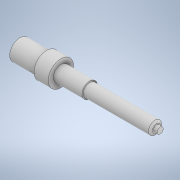
# Autodesk Inventor part: Eixo caixa de engrenagem
Saved by Autodesk Inventor 2022.1 (Build 261234020, 234B)
## iProperties
Created: 2023-11-06
Part Number: Eixo caixa de engrenagem
Material: Generic
Document SubType Name: Modeling
Designer: SENAI
Density: 1 g/cm^3
Appearance: Default
Author: SENAI
Autodesk Inventor part; units mm, degrees
ref_plane "YZ Plane" through (0, 0, 0) normal (1, 0, 0) x (0, 1, 0)
ref_plane "XZ Plane" through (0, 0, 0) normal (0, 1, 0) x (-1, 0, 0)
ref_plane "XY Plane" through (0, 0, 0) normal (0, 0, 1) x (1, 0, 0)
sketch "Sketch1" plane through (0, 0, 0) normal (0, 0, 1) x (1, 0, 0)
  line L0 (0, 0) -> (0, 20)
  line L1 (0, 20) -> (52.5, 20)
  line L2 (52.5, 24.75) -> (80.5, 24.75)
  line L3 (80.5, 15) -> (137, 15)
  line L4 (80.5, 24.75) -> (80.5, 15)
  line L5 (52.5, 24.75) -> (52.5, 20)
  line L6 (137, 12.75) -> (265, 12.75)
  line L7 (137, 12.75) -> (137, 15)
  line L8 (265, 12.75) -> (268, 8.1598)
  line L9 (268, 6) -> (275, 6)
  line L10 (275, 6) -> (275, 0)
  line L11 (268, 8.1598) -> (268, 6)
  line L12 (0, 0) -> (275, 0)
  dimension "d0" = 20
  dimension "d1" = 52.5
  dimension "d3" = 28
  dimension "d5" = 56.5
  dimension "d7" = 128
  dimension "d8" = 131
  dimension "d10" = 7
  dimension "d11" = 33.167
  dimension "d12" = 6.75
  dimension "d13" = 12
  dimension "d14" = 9
  dimension "d15" = 18.75
  constraints: 26 end point, 6 horizontal, 4 vertical, 1 parallel, 1 perpendicular
  measures "d0" distance of L0.start L0.end
  measures "d1" distance of L0.end L1.end
  measures "d3" distance of L2.start L2.end
  measures "d5" distance of L3.start L3.end
  measures "d7" distance of L6.start L6.end
  measures "d8" horizontal distance of L8.end L6.start
  measures "d10" distance of L9.start L9.end
  measures "d11" angle of L10 L8
  measures "d12" distance between parallel lines of L9 L6
  measures "d13" diameter of L9 L12
  measures "d14" distance between parallel lines of L9 L3
  measures "d15" distance between parallel lines of L9 L2
revolve "Revolution1" add sketch "Sketch1" angle 360 about axis through (0, 0, 0) along (1, 0, 0)
body "Solid1"
